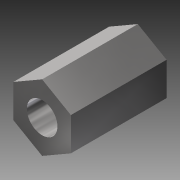
# Autodesk Inventor part: Standoff 40
Saved by Autodesk Inventor 2015 (Build 190159000, 159)
## iProperties
Created: 2016-02-18
Part Number: Standoff 40
Material: Brass, Soft Yellow
Document SubType Name: Modeling
Designer: 23902
Density: 8.47 g/cm^3
Appearance: Brass - Satin
Mass: 1.03642 g
Surface Area: 12.7978 cm^2
Volume: 0.925377 cm^3
Author: 23902
Autodesk Inventor part; units mm, degrees
ref_plane "YZ Plane" through (0, 0, 0) normal (1, 0, 0) x (0, 1, 0)
ref_plane "XZ Plane" through (0, 0, 0) normal (0, 1, 0) x (-1, 0, 0)
ref_plane "XY Plane" through (0, 0, 0) normal (0, 0, 1) x (1, 0, 0)
sketch "Sketch1" plane through (0, 0, 0) normal (0, 1, 0) x (-1, 0, 0)
  circle A0 centre (0, 0) radius 1.6
  line L0 (0, -3.4641) -> (-3, -1.7321)
  line L1 (-3, -1.7321) -> (-3, 1.7321)
  line L2 (-3, 1.7321) -> (0, 3.4641)
  line L3 (0, 3.4641) -> (3, 1.7321)
  line L4 (3, 1.7321) -> (3, -1.7321)
  line L5 (3, -1.7321) -> (0, -3.4641)
  dimension "d0" = 3.2
  dimension "d1" = 6
  constraints: 12 end point, 2 coincident, 1 centre point, 13 other
  measures "d0" diameter of A0
  measures "d1" distance between parallel lines of L0 L3
extrude "Extrusion1" add sketch "Sketch1" along normal blind 10
body "Solid1"
